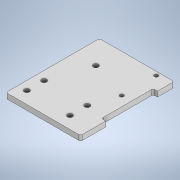
# Autodesk Inventor part: EboxBottom_1
Saved by Autodesk Inventor 2021 (Build 250183000, 183)
## iProperties
Created: 2022-01-03
Part Number: EboxBottom_1
Material: Generic
Document SubType Name: Modeling
Designer: Jorian Brusind
Density: 1 g/cm^3
Appearance: Default
Author: Jorian Brusind
Autodesk Inventor part; units mm, degrees
ref_plane "YZ Plane" through (0, 0, 0) normal (1, 0, 0) x (0, 1, 0)
ref_plane "XZ Plane" through (0, 0, 0) normal (0, 1, 0) x (-1, 0, 0)
ref_plane "XY Plane" through (0, 0, 0) normal (0, 0, 1) x (1, 0, 0)
sketch "Sketch1" plane through (0, 0, 0) normal (0, 1, 0) x (-1, 0, 0)
  line L0 (232.1908, -176.5808) -> (232.1908, -3.7592)
  arc A0 (232.1908, -3.7592) -> (227.4316, 1) centre (227.4316, -3.7592) ccw
  line L1 (227.4316, 1) -> (0, 1)
  arc A1 (0, 1) -> (-4.7592, -3.7592) centre (0, -3.7592) ccw
  arc A2 (-4.7592, -176.5808) -> (0, -181.34) centre (0, -176.5808) ccw
  arc A3 (227.4316, -181.34) -> (232.1908, -176.5808) centre (227.4316, -176.5808) ccw
  circle A4 centre (130, -135) radius 2.25
  circle A5 centre (130, -95) radius 2.25
  circle A6 centre (90, -135) radius 2.25
  circle A7 centre (90, -95) radius 2.25
  circle A8 centre (175, -110) radius 3
  circle A9 centre (55, -110) radius 3
  circle A10 centre (90, -45) radius 3
  circle A11 centre (190, -45) radius 3
  circle A12 centre (190, -65) radius 3
  circle A13 centre (90, -65) radius 3
  circle A14 centre (140, -45) radius 3
  circle A15 centre (40, -45) radius 3
  circle A16 centre (140, -65) radius 3
  circle A17 centre (40, -65) radius 3
  line L2 (230.1908, -176.5808) -> (230.1908, -3.7592)
  arc A18 (230.1908, -3.7592) -> (227.4316, -1) centre (227.4316, -3.7592) ccw
  line L3 (227.4316, -1) -> (0, -1)
  arc A19 (0, -1) -> (-2.7592, -3.7592) centre (0, -3.7592) ccw
  arc A20 (-2.7592, -176.5808) -> (0, -179.34) centre (0, -176.5808) ccw
  arc A21 (227.4316, -179.34) -> (230.1908, -176.5808) centre (227.4316, -176.5808) ccw
  line L4 (-4.7592, -3.7592) -> (-4.7592, -176.5808)
  line L5 (-2.7592, -3.7592) -> (-2.7592, -176.5808)
  line L6 (0, -179.34) -> (227.4316, -179.34)
  line L7 (227.4316, -181.34) -> (0, -181.34)
  line L8 (0, 0) -> (0, -15)
  line L9 (0, 0) -> (15, 0) construction
  line L10 (0, 0) -> (15, 0)
  line L11 (0, 0) -> (15, 0) construction
  point P0 (230.1908, -3.7592)
  point P1 (0, -1)
  dimension "d0" = 2
  dimension "d1" = 2
  dimension "d2" = 2
  dimension "d3" = 2
  dimension "d5" = 2
  dimension "d7" = 2
  dimension "d8" = 227.4316
  dimension "d9" = 172.8216
  dimension "d10" = 4.7592
  dimension "d45" = 15
  dimension "d46" = 90
  dimension "d47" = 15
  dimension "d48" = 0
  dimension "d49" = 55
  dimension "d50" = 110
  dimension "d51" = 120
  dimension "d52" = 110
  dimension "d54" = 6
  dimension "d55" = 6
  dimension "d56" = 4.5
  dimension "d57" = 6
  dimension "d58" = 6
  dimension "d59" = 6
  dimension "d60" = 6
  dimension "d61" = 6
  dimension "d62" = 6
  dimension "d63" = 6
  dimension "d64" = 6
  dimension "d65" = 4.5
  dimension "d66" = 4.5
  dimension "d67" = 4.5
  constraints: 24 end point, 22 centre point, 16 point on circle, 7 equal length, 3 horizontal, 2 vertical, 1 tangent
  measures "d0" distance between parallel lines of L0 L2
  measures "d1" radial gap between concentric circles of A0 A18
  measures "d2" distance between parallel lines of L1 L3
  measures "d3" radial gap between concentric circles of A1 A19
  measures "d5" radial gap between concentric circles of A2 A20
  measures "d7" radial gap between concentric circles of A3 A21
  measures "d8" distance of L7.start L7.end
  measures "d9" distance of L0.start L0.end
  measures "d10" radius of A3
  measures "d45" distance of L8.start L8.end
  measures "d46" angle of L8 L9
  measures "d47" distance of L8.start L9.end
  measures "d48" distance between parallel lines of L10 L11
  measures "d49" distance from line of A9.centre L8
  measures "d50" distance from line of L9 A9.centre
  measures "d51" distance of A9.centre A8.centre
  measures "d52" distance from line of L9 A8.centre
  measures "d54" diameter of A8
  measures "d55" diameter of A9
  measures "d56" diameter of A6
  measures "d57" diameter of A12
  measures "d58" diameter of A11
  measures "d59" diameter of A14
  measures "d60" diameter of A16
  measures "d61" diameter of A13
  measures "d62" diameter of A17
  measures "d63" diameter of A15
  measures "d64" diameter of A10
  measures "d65" diameter of A4
  measures "d66" diameter of A5
  measures "d67" diameter of A7
extrude "Extrusion1" add sketch "Sketch1" along normal blind 6 contours A21 L6 A20 L5 A19 L3 A18 L2
sketch "Sketch2" plane through (0, 6, 0) normal (0, 1, 0) x (1, 0, 0)
  line L0 (-232.1908, 176.5808) -> (-232.1908, 3.7592)
  arc A0 (-232.1908, 3.7592) -> (-227.4316, -1) centre (-227.4316, 3.7592) ccw
  line L1 (-227.4316, -1) -> (0, -1)
  arc A1 (0, -1) -> (4.7592, 3.7592) centre (0, 3.7592) ccw
  arc A2 (4.7592, 176.5808) -> (0, 181.34) centre (0, 176.5808) ccw
  arc A3 (-227.4316, 181.34) -> (-232.1908, 176.5808) centre (-227.4316, 176.5808) ccw
  circle A4 centre (-130, 135) radius 2
  circle A5 centre (-130, 95) radius 2
  circle A6 centre (-90, 135) radius 2
  circle A7 centre (-90, 95) radius 2
  circle A8 centre (-160.0797, 100) radius 2.75
  circle A9 centre (-60.0797, 100) radius 2.75
  circle A10 centre (-90, 45) radius 2.5
  circle A11 centre (-190, 45) radius 2.5
  circle A12 centre (-190, 65) radius 2.5
  circle A13 centre (-90, 65) radius 2.5
  circle A14 centre (-140, 45) radius 2.5
  circle A15 centre (-40, 45) radius 2.5
  circle A16 centre (-140, 65) radius 2.5
  circle A17 centre (-40, 65) radius 2.5
  line L2 (-230.1908, 176.5808) -> (-230.1908, 3.7592)
  arc A18 (-230.1908, 3.7592) -> (-227.4316, 1) centre (-227.4316, 3.7592) ccw
  line L3 (-227.4316, 1) -> (0, 1)
  arc A19 (0, 1) -> (2.7592, 3.7592) centre (0, 3.7592) ccw
  arc A20 (2.7592, 176.5808) -> (0, 179.34) centre (0, 176.5808) ccw
  arc A21 (-227.4316, 179.34) -> (-230.1908, 176.5808) centre (-227.4316, 176.5808) ccw
  line L4 (4.7592, 3.7592) -> (4.7592, 176.5808)
  line L5 (2.7592, 3.7592) -> (2.7592, 176.5808)
  line L6 (0, 179.34) -> (-227.4316, 179.34)
  line L7 (-227.4316, 181.34) -> (0, 181.34)
  line L8 (0, 179.34) -> (-227.4316, 179.34) projected
  line L9 (-113.7158, 179.34) -> (-113.7158, 1)
  line L10 (-227.4316, 1) -> (0, 1) projected
  line L11 (-118.7158, 120.17) -> (-108.7158, 120.17)
  line L12 (-108.7158, 120.17) -> (-108.7158, 60.17)
  line L13 (-108.7158, 60.17) -> (-118.7158, 60.17)
  line L14 (-118.7158, 60.17) -> (-118.7158, 120.17)
  line L15 (-118.7158, 120.17) -> (-108.7158, 60.17) construction
  line L16 (-108.7158, 120.17) -> (-118.7158, 60.17) construction
  line L17 (-113.7158, 179.34) -> (-113.7158, 159.34)
  line L18 (2.7592, 139.34) -> (-230.1908, 139.34)
  line L19 (-230.1908, 139.34) -> (-230.1908, 179.34)
  line L20 (-230.1908, 179.34) -> (2.7592, 179.34)
  line L21 (2.7592, 179.34) -> (2.7592, 139.34)
  line L22 (2.7592, 139.34) -> (-230.1908, 179.34) construction
  line L23 (-230.1908, 139.34) -> (2.7592, 179.34) construction
  line L24 (-113.7158, 1) -> (-113.7158, 16)
  line L25 (-230.1908, 31) -> (2.7592, 31)
  line L26 (2.7592, 31) -> (2.7592, 1)
  line L27 (2.7592, 1) -> (-230.1908, 1)
  line L28 (-230.1908, 1) -> (-230.1908, 31)
  line L29 (-230.1908, 31) -> (2.7592, 1) construction
  line L30 (2.7592, 31) -> (-230.1908, 1) construction
  line L31 (-227.4316, 1) -> (0, 1) projected
  line L32 (-230.1908, 179.34) -> (-200.1908, 179.34)
  line L33 (-200.1908, 179.34) -> (-200.1908, 1)
  line L34 (-200.1908, 1) -> (-230.1908, 1)
  line L35 (-230.1908, 1) -> (-230.1908, 179.34)
  line L36 (2.7592, 1) -> (-27.2408, 1)
  line L37 (-27.2408, 1) -> (-27.2408, 179.34)
  line L38 (-27.2408, 179.34) -> (2.7592, 179.34)
  line L39 (2.7592, 179.34) -> (2.7592, 1)
  line L40 (-200.1908, 139.34) -> (-113.7158, 139.34)
  point P0 (230.1908, -176.5808)
  point P1 (230.1908, -3.7592)
  point P2 (227.4316, -1)
  point P3 (0, -1)
  point P4 (0, 0)
  point P5 (230.1908, -176.5808)
  point P6 (230.1908, -3.7592)
  point P7 (227.4316, -1)
  point P8 (0, -1)
  point P9 (-113.7158, 90.17)
  point P10 (-113.7158, 120.17)
  point P11 (-113.7158, 60.17)
  point P12 (-113.7158, 1)
  point P13 (0, 1)
  point P14 (-113.7158, 139.34)
  point P15 (-113.7158, 31)
  point P16 (-200.1908, 31)
  point P17 (-230.1908, 3.7592)
  point P18 (-227.4316, 1)
  dimension "d22" = 2
  dimension "d23" = 2
  dimension "d24" = 2
  dimension "d25" = 2
  dimension "d26" = 2
  dimension "d27" = 2
  dimension "d28" = 227.4316
  dimension "d29" = 172.8216
  dimension "d30" = 4.7592
  dimension "d31" = 10
  dimension "d32" = 60
  dimension "d37" = 20
  dimension "d38" = 40
  dimension "d39" = 15
  dimension "d40" = 30
  dimension "d41" = 30
  dimension "d42" = 30
  constraints: 76 end point, 22 centre point, 16 point on circle, 14 parallel, 10 midpoint, 6 point on line, 5 horizontal, 5 perpendicular, 1 tangent
  measures "d22" distance between parallel lines of L0 L2
  measures "d23" radial gap between concentric circles of A0 A18
  measures "d24" distance between parallel lines of L1 L3
  measures "d25" radial gap between concentric circles of A1 A19
  measures "d26" radial gap between concentric circles of A2 A20
  measures "d27" radial gap between concentric circles of A3 A21
  measures "d28" distance of L7.start L7.end
  measures "d29" distance of L0.start L0.end
  measures "d30" radius of A3
  measures "d31" distance of L12.end L13.end
  measures "d32" distance of L11.end L12.end
  measures "d37" distance of L9.start L17.end
  measures "d38" distance of L18.end L19.end
  measures "d39" distance of L9.end L24.end
  measures "d40" distance of L25.end L26.end
  measures "d41" distance of L33.end L34.end
  measures "d42" distance of L37.end L38.end
extrude "Extrusion3" cut sketch "Sketch2" against normal through all contours A6 | A7 | A9 | A10 | A13 | A15 | A17 | A21 L6 L33 L18 L2 | L18 L33 L25 L2 | L25 L33 L3 A18 L2 | L33 L6 L9 L18 | L25 L9 L3 L33 | L18 L37 L25 L9 L13 L12 L11 | L9 L6 L37 L18 | L25 L37 L3 L9 | L11 L12 L13 L9 | L9 L13 L14 L11 | L37 L6 A20 L5 L18 | L18 L5 L25 L37 | L25 L5 A19 L3 L37
fillet "Fillet3" radius 2 6 edges at (-113.7158, 3, -31) (-200.1908, 3, -31) (-113.7158, 3, -139.34) (-118.7158, 3, -120.17) (-118.7158, 3, -60.17) (-200.1908, 3, -139.34)
equation "\"d1\" = d0"
equation "\"d2\" = d0"
equation "\"d3\" = d0"
equation "\"d5\" = d0"
equation "\"d7\" = d0"
equation "\"d23\" = d22"
equation "\"d24\" = d22"
equation "\"d25\" = d22"
equation "\"d26\" = d22"
equation "\"d27\" = d22"
body "Solid1"
